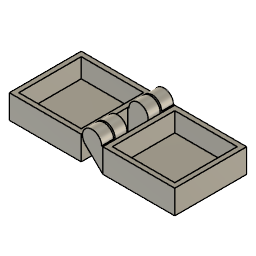
Oct30_Hinge (Autodesk Fusion 360 design; units mm, degrees)
part number: 2025-10-30-22-06-32-350
part number: 2025-10-30-22-06-37-722
part number: 2025-10-30-22-07-04-902
Autodesk Fusion 360 part; units mm, degrees
sketch "Box Width" plane through (0, 0, 0) normal (0, 0, 1) x (1, 0, 0) in component "BoxTop"
  line L0 (0, 0) -> (-30, 0)
  line L1 (-30, 0) -> (-30, -30)
  line L2 (-30, -30) -> (0, -30)
  line L3 (0, -30) -> (0, 0)
  dimension "d3_1" = 30
  dimension "d4_1" = 30
  constraint horizontal L0
  constraint vertical L1
  constraint horizontal L2
  constraint vertical L3
  constraint coincident L0.start L3.end
  measures "d3_1" distance of L0.start L0.end
  measures "d4_1" distance of L0.start L2.end
extrude "Extrude1" add sketch "Box Width" along normal blind 10 makes body 1 in component "BoxTop"
shell "Shell1" thickness 2 removed faces 1 at (-20, -10, 10) on bodies 1 in component "BoxTop"
sketch "Box Width (2)" plane through (0, 0, 0) normal (0, 0, 1) x (1, 0, 0) in component "BoxBottom (1)"
  line L0 (0, 0) -> (-30, 0)
  line L1 (-30, 0) -> (-30, -30)
  line L2 (-30, -30) -> (0, -30)
  line L3 (0, -30) -> (0, 0)
  dimension "d3_2" = 30
  dimension "d4_2" = 30
  constraint horizontal L0
  constraint vertical L1
  constraint horizontal L2
  constraint vertical L3
  constraint coincident L0.start L3.end
  measures "d3_2" distance of L0.start L0.end
  measures "d4_2" distance of L0.start L2.end
extrude "Extrude1'" add sketch "Box Width (2)" along normal blind 10 separate body makes body 2 in component "BoxBottom (1)"
shell "Shell1'" thickness 2 removed faces 1 at (-20, -10, 10) on bodies 2 in component "BoxBottom (1)"
sketch "Sketch1" plane through (0, -30, 0) normal (0, -1, 0) x (1, 0, 0)
  line L0 (-30, 0) -> (0, 0)
  line L1 (0, 0) -> (0, 10)
  line L2 (0, 10) -> (-30, 10)
  line L3 (-30, 10) -> (-30, 0)
  line L4 (-30, 10) -> (-34.5, 10)
  circle A0 centre (-34.5, 10) radius 4
  line L5 (-30, 0) -> (-37.2976, 7.1411)
  dimension "d5" = 4.5
  dimension "d6" = 8
  constraint coincident L2.end L3.start
  constraint perpendicular L3 L4
  constraint coincident L4.end A0.centre
  constraint coincident L0.start L3.end
  constraint coincident A0 L5.end
  constraint tangent A0 L5
  measures "d5" distance of L2.end L4.end
  measures "d6" diameter of A0
extrude "Extrude1''" add sketch "Sketch1" against normal blind 5 separate body contours L3 L4 A0 L5 | A0 makes body 3
sketch "Sketch2" plane through (0, -25, 0) normal (0, 1, 0) x (-1, 0, 0)
  line L0 (30.5, 10) -> (30, 10)
  line L1 (30, 10) -> (30, 0)
  line L2 (30, 0) -> (37.2976, 7.1411)
  arc A0 (37.2976, 7.1411) -> (30.5, 10) centre (34.5, 10) ccw
  arc A1 (37.2976, 7.1411) -> (30.5, 10) centre (34.5, 10) ccw
  circle A2 centre (34.5, 10) radius 2
  dimension "d9" = 4
  constraint concentric A1 A2
  measures "d9" diameter of A2
extrude "Extrude2" add sketch "Sketch2" along normal blind 3.8 draft -14 contours A2 bodies 3
sketch "Sketch3" plane through (0, -25, 0) normal (0, 1, 0) x (-1, 0, 0)
  circle A0 centre (34.5, 10) radius 2
  line L0 (30.5, 10) -> (30, 10)
  line L1 (30, 10) -> (30, 0)
  line L2 (30, 0) -> (37.2976, 7.1411)
  arc A1 (37.2976, 7.1411) -> (30.5, 10) centre (34.5, 10) ccw
  line L3 (39, 10) -> (38.5, 10)
  circle A2 centre (34.5, 10) radius 4
  line L4 (39, 0) -> (31.7024, 7.1411)
  line L5 (39, 0) -> (39, 10)
  constraint coincident A1 L3.end
  constraint horizontal L3
  constraint concentric A0 A2
  constraint coincident A2 L4.end
  constraint tangent A2 L4
extrude "Extrude3" add sketch "Sketch3" along normal blind 5 from surface at 0.6 separate body contours A0 | A1 A2 | L2 A1 L3 A2 L4 L5 | L2 A2 L4 makes body 4
combine "Combine1" operation cut target body 4 tool bodies 3 keep tools
move_face "OffsetFaces1" offset -0.4 2 faces at (-34.2272, -21.2, 10.3421) (-34.3717, -23.8667, 11.7126) on bodies 4
ref_plane "WorkPlane1" through (-15, -15, 5) normal (0, -1, 0) x (1, 0, 0)
mirror "Mirror1" about plane through (-15, -15, 5) normal (0, -1, 0) of bodies 4 makes body 5
mirror "Mirror2" about plane through (-15, -15, 5) normal (0, -1, 0) of bodies 3 makes body 6
component "BoxTop" placed x (0, 1, 0) y (-1, 0, 0) z (0, 0, 1) at (-69, 0, 0)
component "BoxBottom (1)" placed x (1, 0, 0) y (0, 1, 0) z (0, 0, 1) at (0, 0, 0)
equation "d3_1 = Boxwidth_1"
equation "d4_1 = Boxwidth_1"
equation "d5_1 = Boxheight_1 / 2"
equation "Wallthickness_1 = 2 mm"
equation "Boxwidth_1 = 30 mm"
equation "Boxheight_1 = 20 mm"
equation "d3_2 = Boxwidth_2"
equation "d4_2 = Boxwidth_2"
equation "d5_2 = Boxheight_2 / 2"
equation "Wallthickness_2 = 2 mm"
equation "Boxwidth_2 = 30 mm"
equation "Boxheight_2 = 20 mm"
